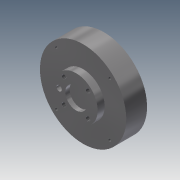
# Autodesk Inventor part: HandMountingFlange
Saved by Autodesk Inventor 2015 (Build 190159000, 159)
## iProperties
Created: 2016-10-09
Part Number: HandMountingFlange
Material: PAEK 樹脂
Document SubType Name: Modeling
Designer: tAkaharu
Density: 1.32 g/cm^3
Appearance: ステンレス - ブラシ仕上げ
Author: tAkaharu
Autodesk Inventor part; units mm, degrees
ref_plane "YZ Plane" through (0, 0, 0) normal (1, 0, 0) x (0, 1, 0)
ref_plane "XZ Plane" through (0, 0, 0) normal (0, 1, 0) x (-1, 0, 0)
ref_plane "XY Plane" through (0, 0, 0) normal (0, 0, 1) x (1, 0, 0)
sketch "スケッチ1" plane through (0, 0, 0) normal (0, 1, 0) x (-1, 0, 0)
  circle A0 centre (0, 0) radius 40
  dimension "d0" = 80
  constraints: 1 centre point, 1 coincident
  measures "d0" diameter of A0
extrude "押し出し1" add sketch "スケッチ1" along normal blind 19.3
sketch "スケッチ3" plane through (0, 19.3, 0) normal (0, 1, 0) x (1, 0, 0)
  circle A0 centre (0, 0) radius 20
  dimension "d3" = 40
  constraints: 1 centre point, 1 coincident
  measures "d3" diameter of A0
extrude "押し出し2" add sketch "スケッチ3" along normal blind 6.5
sketch "スケッチ4" plane through (0, 25.8, 0) normal (0, 1, 0) x (1, 0, 0)
  circle A0 centre (0, 0) radius 10
  dimension "d6" = 20
  constraints: 1 centre point, 1 coincident
  measures "d6" diameter of A0
extrude "押し出し3" cut sketch "スケッチ4" against normal blind 4
sketch "スケッチ5" plane through (0, 19.3, 0) normal (0, 1, 0) x (1, 0, 0)
  point P0 (0, 0)
  point P1 (0, 0)
  point P2 (-24.7487, -24.7487)
  point P3 (24.7487, -24.7487)
  point P4 (24.7487, 24.7487)
  point P5 (-24.7487, 24.7487)
  dimension "d9" = 35
  dimension "d12" = 360
  constraints: 1 coincident, 5 other
  measures "d9" distance of point (0, 0) point (-24.749, -24.749)
hole "穴1" at (-24.7487, 19.3, -24.7487) at (-24.7487, 19.3, 24.7487) at (24.7487, 19.3, 24.7487) at (24.7487, 19.3, -24.7487) direction (0, -1, 0) diameter 2.459 depth 6 tip angle 118 thread size "M3x0.5" class "6H" standard "ANSI Metric M Profile"
sketch "スケッチ6" plane through (0, 25.8, 0) normal (0, 1, 0) x (1, 0, 0)
  point P0 (0, 0)
  point P1 (-11.1369, -11.1369)
  point P2 (11.1369, -11.1369)
  point P3 (11.1369, 11.1369)
  point P4 (-11.1369, 11.1369)
  dimension "d21" = 15.75
  dimension "d24" = 360
  constraints: 5 other
  measures "d21" distance of point (-11.137, -11.137) point (0, 0)
hole "穴2" at (-11.1369, 25.8, 11.1369) at (11.1369, 25.8, 11.1369) at (11.1369, 25.8, -11.1369) at (-11.1369, 25.8, -11.1369) direction (0, -1, 0) diameter 4.134 depth 8 tip angle 118 thread size "M5x0.8" class "6H" standard "ANSI Metric M Profile"
sketch "スケッチ7" plane through (0, 25.8, 0) normal (0, 1, 0) x (1, 0, 0)
  point P0 (0, 0)
  point P1 (0, 15.75)
  dimension "d33" = 15.75
  measures "d33" distance of point (0, 0) point (0, 15.75)
hole "穴3" at (0, 25.8, -15.75) direction (0, -1, 0) diameter 5 depth 8 tip angle 118
sketch "スケッチ8" plane through (0, 0, 0) normal (0, -1, 0) x (1, 0, 0)
  circle A0 centre (0, 0) radius 5
  dimension "d41" = 10
  constraints: 1 centre point, 1 coincident
  measures "d41" diameter of A0
extrude "押し出し4" cut sketch "スケッチ8" against normal blind 10
move or copy body "ボディを移動2" bodies to move or copy 1 copy no rotation origin (0, 0, 0) rotation axis (1, 0, 0) rotation angle 90
move or copy body "ボディを移動3" bodies to move or copy 1 copy no rotation origin (0, 0, 0) rotation axis (0, 0, 1) rotation angle 90
